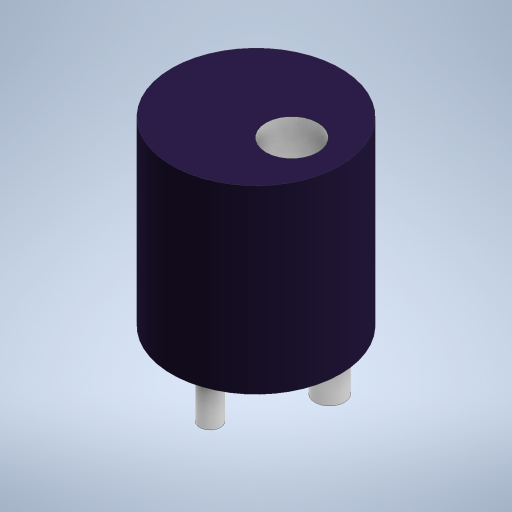
# Autodesk Inventor part: Conector de carga
Saved by Autodesk Inventor 2024 (Build 280153000, 153)
## iProperties
Created: 2024-05-05
Part Number: Conector de carga
Material: Generic
Document SubType Name: Modeling
Designer: samue
Density: 1 g/cm^3
Appearance: Default
Author: samue
Autodesk Inventor part; units mm, degrees
ref_plane "YZ Plane" through (0, 0, 0) normal (1, 0, 0) x (0, 1, 0)
ref_plane "XZ Plane" through (0, 0, 0) normal (0, 1, 0) x (-1, 0, 0)
ref_plane "XY Plane" through (0, 0, 0) normal (0, 0, 1) x (1, 0, 0)
sketch "Sketch1" plane through (0, 0, 0) normal (0, 1, 0) x (-1, 0, 0)
  circle A0 centre (0, 0) radius 7
  dimension "d0" = 14
  constraints: 1 centre point, 1 coincident
  measures "d0" diameter of A0
extrude "Extrusion1" add sketch "Sketch1" along normal blind 15
sketch "Sketch2" plane through (0, 15, 0) normal (0, 1, 0) x (1, 0, 0)
  circle A0 centre (2.9736, 0) radius 2.141
  point P0 (0, 0)
  constraints: 1 centre point
extrude "Extrusion2" cut sketch "Sketch2" against normal blind 10
sketch "Sketch3" plane through (0, 0, 0) normal (0, -1, 0) x (1, 0, 0)
  circle A0 centre (0, 3.8062) radius 0.8659
  circle A1 centre (2.9736, -3.1401) radius 1.2343
  circle A2 centre (-2.7357, -2.141) radius 0.6471
  point P0 (0, 0)
  constraints: 3 centre point
extrude "Extrusion3" add sketch "Sketch3" along normal blind 5
body "Solid1"
